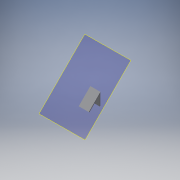
# Autodesk Inventor part: Support
Saved by Autodesk Inventor 2017 (Build 210142000, 142)
## iProperties
Created: 2017-01-19
Part Number: Support
Material: Generic
Document SubType Name: Modeling
Designer: kingb
Density: 1 g/cm^3
Appearance: Default
Author: kingb
Autodesk Inventor part; units mm, degrees
ref_plane "YZ Plane" through (0, 0, 0) normal (1, 0, 0) x (0, 1, 0)
ref_plane "XZ Plane" through (0, 0, 0) normal (0, 1, 0) x (-1, 0, 0)
ref_plane "XY Plane" through (0, 0, 0) normal (0, 0, 1) x (1, 0, 0)
ref_plane "Work Plane1" through (85.725, 80.736, -75.2679) normal (-1, 0, 0) x (0, -0.704501, -0.709703)
sketch "Sketch1" plane through (85.725, 80.736, -75.2679) normal (-1, 0, 0) x (0, -0.704501, -0.709703)
  line L0 (3.4608, 0) -> (3.4607, 241.3) projected
  line L1 (5.6975, 112.5782) -> (38.7126, 145.837) projected
  line L2 (3.4608, 110.3249) -> (5.6975, 112.5782) projected
  line L3 (38.7126, 145.837) -> (36.4593, 148.0738)
  line L4 (36.4593, 148.0738) -> (6.6358, 118.0301)
  line L5 (6.6358, 118.0301) -> (6.6358, 177.6787)
  line L6 (6.6358, 177.6787) -> (3.4607, 177.6787)
  line L7 (3.4607, 177.6787) -> (3.4608, 110.3249)
  line L8 (3.4608, 110.3249) -> (38.7126, 145.837)
  dimension "d0" = 3.175
  dimension "d1" = 3.175
  constraints: 12 end point, 2 collinear, 2 perpendicular, 1 point on line
  measures "d0" distance of L1.end L3.end
  measures "d1" distance from line of L0 L4.end
extrude "Extrusion1" add sketch "Sketch1" against normal blind 41.275
body "Solid1"
